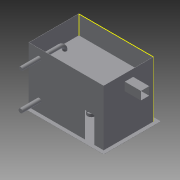
# Autodesk Inventor part: LLNL_Enclosure_Drawing
Saved by Autodesk Inventor 2013 SP2 (Build 170200200, 200)
## iProperties
Created: 2014-01-13
Part Number: LLNL_Enclosure_Drawing
Material: Generic
Document SubType Name: Modeling
Designer: mcgratta
Density: 1 g/cm^3
Author: mcgratta
Autodesk Inventor part; units mm, degrees
ref_plane "YZ Plane" through (0, 0, 0) normal (1, 0, 0) x (0, 1, 0)
ref_plane "XZ Plane" through (0, 0, 0) normal (0, 1, 0) x (-1, 0, 0)
ref_plane "XY Plane" through (0, 0, 0) normal (0, 0, 1) x (1, 0, 0)
sketch "Sketch1" plane through (0, 0, 0) normal (0, 1, 0) x (-1, 0, 0)
  line L0 (0, 0) -> (-6600, 0)
  line L1 (-6600, 0) -> (-6600, -4600)
  line L2 (-6600, -4600) -> (0, -4600)
  line L3 (0, -4600) -> (0, 0)
  dimension "d0" = 6600
  dimension "d2" = 4600
  constraints: 8 end point, 2 parallel, 1 horizontal, 1 perpendicular
  measures "d0" distance of L1.end L2.end
  measures "d2" distance of L2.end L0.start
extrude "Extrusion1" add sketch "Sketch1" along normal blind 10
sketch "Sketch2" plane through (0, 10, 0) normal (0, 1, 0) x (1, 0, 0)
  line L0 (0, 0) -> (6600, 0) projected
  line L1 (6600, 0) -> (6600, 4600) projected
  line L2 (6600, 4600) -> (0, 4600) projected
  line L3 (0, 4600) -> (0, 0) projected
  line L4 (300, 4300) -> (6300, 4300)
  line L5 (6300, 4300) -> (6300, 300)
  line L6 (6300, 300) -> (300, 300)
  line L7 (300, 300) -> (300, 4300)
  line L8 (280, 4320) -> (6320, 4320)
  line L9 (6320, 4320) -> (6320, 280)
  line L10 (6320, 280) -> (280, 280)
  line L11 (280, 280) -> (280, 4320)
  dimension "d5" = 300
  dimension "d6" = 300
  dimension "d7" = 300
  dimension "d8" = 300
  dimension "d9" = 20
  dimension "d10" = 20
  dimension "d11" = 20
  dimension "d12" = 20
  constraints: 16 end point, 4 parallel, 2 horizontal, 2 perpendicular
  measures "d5" distance between parallel lines of L7 L3
  measures "d6" distance between parallel lines of L4 L2
  measures "d7" distance between parallel lines of L1 L5
  measures "d8" distance between parallel lines of L0 L6
  measures "d9" distance between parallel lines of L7 L11
  measures "d10" distance between parallel lines of L4 L8
  measures "d11" distance between parallel lines of L6 L10
  measures "d12" distance between parallel lines of L5 L9
extrude "Extrusion2" add sketch "Sketch2" along normal blind 4500 contours L8 L9 L10 L11
sketch "Sketch3" plane through (280, 10, -280) normal (0, 0, 1) x (1, 0, 0)
  line L0 (6040, 0) -> (0, 0) projected
  line L1 (6040, 0) -> (6040, 4500) projected
  line L2 (4530, 0) -> (5290, 0)
  line L3 (5290, 0) -> (5290, 2060)
  line L4 (5290, 2060) -> (4530, 2060)
  line L5 (4530, 2060) -> (4530, 0)
  point P0 (-280, -10)
  dimension "d15" = 750
  dimension "d16" = 760
  dimension "d17" = 2060
  constraints: 8 end point, 2 parallel, 1 horizontal, 1 perpendicular, 1 point on line
  measures "d15" distance between parallel lines of L1 L3
  measures "d16" distance between parallel lines of L3 L5
  measures "d17" distance between parallel lines of L0 L4
extrude "Extrusion3" cut sketch "Sketch3" along normal mid plane 40
sketch "Sketch4" plane through (300, 10, -4300) normal (0, 0, 1) x (1, 0, 0)
  line L0 (6000, 0) -> (0, 0) projected
  line L1 (6000, 0) -> (6000, 4500) projected
  line L2 (0, 4500) -> (6000, 4500) projected
  line L3 (0, 0) -> (0, 4500) projected
  point P0 (-300, -10)
sketch "Sketch5" plane through (300, 10, -4300) normal (0, 0, 1) x (1, 0, 0)
  line L0 (6000, 0) -> (6000, 4500) projected
  line L1 (0, 4500) -> (6000, 4500) projected
  line L2 (0, 0) -> (0, 4500) projected
  line L3 (0, 3000) -> (6000, 3000)
  line L4 (6000, 3000) -> (6000, 2980)
  line L5 (6000, 2980) -> (0, 2980)
  line L6 (0, 2980) -> (0, 3000)
  point P0 (-300, -10)
  dimension "d20" = 1500
  dimension "d21" = 20
  constraints: 8 end point, 2 parallel, 2 point on line, 1 horizontal, 1 perpendicular
  measures "d20" distance between parallel lines of L3 L1
  measures "d21" distance between parallel lines of L5 L3
extrude "Extrusion4" add sketch "Sketch5" along normal up to next contours L5 L2 L3 L0
sketch "Sketch7" plane through (300, 3010, -4300) normal (0, 1, 0) x (1, 0, 0)
  line L0 (6000, -4000) -> (0, -4000) projected
  line L1 (6000, 0) -> (6000, -4000) projected
  line L2 (5200, -1800) -> (5600, -1800)
  line L3 (5600, -1800) -> (5600, -2200)
  line L4 (5600, -2200) -> (5200, -2200)
  line L5 (5200, -2200) -> (5200, -1800)
  point P0 (-300, -4300)
  dimension "d31" = 400
  dimension "d33" = 400
  dimension "d34" = 1800
  dimension "d35" = 400
  constraints: 8 end point, 2 parallel, 1 horizontal, 1 perpendicular
  measures "d31" distance between parallel lines of L3 L5
  measures "d33" distance between parallel lines of L2 L4
  measures "d34" distance between parallel lines of L0 L4
  measures "d35" distance between parallel lines of L1 L3
extrude "Extrusion6" cut sketch "Sketch7" along normal mid plane 40
sketch "Sketch8" plane through (280, 4510, -280) normal (0, 0, 1) x (1, 0, 0)
  circle A0 centre (850, -669.704) radius 150
  line L0 (0, -4500) -> (0, 0) projected
  point P0 (-280, -4510)
  dimension "d38" = 300
  dimension "d70" = 850
  constraints: 1 centre point
  measures "d38" diameter of A0
  measures "d70" distance from line of A0.centre L0
extrude "Extrusion7" add sketch "Sketch8" along normal blind 1500 and the other way blind 1600
sketch "Sketch9" plane through (1130, 3840.296, -1880) normal (0, 0, -1) x (-1, 0, 0)
  circle A0 centre (0, 0) radius 150 projected
  circle A1 centre (0, 0) radius 150
  line L0 (150, -467.722) -> (-150, -467.722)
  point P0 (1130, -3840.296)
  dimension "d44" = 300
  constraints: 2 end point, 1 centre point, 1 coincident, 1 concentric, 1 horizontal
  measures "d44" diameter of A1
revolve "Revolution1" add sketch "Sketch9" angle 90 about axis through (980, 3372.574, -1880) along (-1, 0, 0)
sketch "Sketch10" plane through (6320, 10, -280) normal (1, 0, 0) x (0, 0, -1)
  line L0 (4040, 0) -> (0, 0) projected
  line L1 (4040, 0) -> (4040, 4500) projected
  line L2 (1715, 3925) -> (2365, 3925)
  line L3 (2365, 3925) -> (2365, 3275)
  line L4 (2365, 3275) -> (1715, 3275)
  line L5 (1715, 3275) -> (1715, 3925)
  line L6 (1705, 3935) -> (2375, 3935)
  line L7 (2375, 3935) -> (2375, 3265)
  line L8 (2375, 3265) -> (1705, 3265)
  line L9 (1705, 3265) -> (1705, 3935)
  point P0 (-280, -10)
  dimension "d46" = 650
  dimension "d48" = 650
  dimension "d49" = 3275
  dimension "d50" = 1675
  dimension "d51" = 10
  dimension "d52" = 10
  dimension "d53" = 10
  dimension "d54" = 10
  constraints: 16 end point, 4 parallel, 2 horizontal, 2 perpendicular
  measures "d46" distance between parallel lines of L3 L5
  measures "d48" distance between parallel lines of L4 L2
  measures "d49" distance between parallel lines of L0 L4
  measures "d50" distance between parallel lines of L1 L3
  measures "d51" distance between parallel lines of L2 L6
  measures "d52" distance between parallel lines of L5 L9
  measures "d53" distance between parallel lines of L4 L8
  measures "d54" distance between parallel lines of L3 L7
extrude "Extrusion9" add sketch "Sketch10" along normal blind 1300
sketch "Sketch11" plane through (0, 10, 0) normal (0, 1, 0) x (1, 0, 0)
  line L0 (0, 0) -> (6600, 0) projected
  line L1 (0, 4600) -> (0, 0) projected
  circle A0 centre (3300, 2300) radius 285
  circle A1 centre (3300, 2300) radius 300
  dimension "d59" = 570
  dimension "d61" = 2300
  dimension "d62" = 3300
  dimension "d63" = 600
  constraints: 2 centre point, 1 coincident
  measures "d59" diameter of A0
  measures "d61" distance from line of L0 A0.centre
  measures "d62" distance from line of L1 A0.centre
  measures "d63" diameter of A1
extrude "Extrusion10" add sketch "Sketch11" along normal blind 230
sketch "Sketch12" plane through (280, 4510, -280) normal (0, 0, 1) x (1, 0, 0)
  circle A0 centre (850, -3599.0075) radius 161.8593
  line L0 (0, -4500) -> (0, 0) projected
  point P0 (-280, -4510)
  dimension "d71" = 850
  constraints: 1 centre point
  measures "d71" distance from line of L0 A0.centre
extrude "Extrusion11" add sketch "Sketch12" along normal blind 1500 and the other way blind 1500
body "Solid1"
